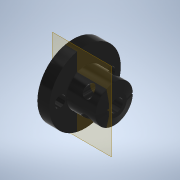
# Autodesk Inventor part: Hub
Saved by Autodesk Inventor 2022 (Build 260153000, 153)
## iProperties
Created: 2022-07-25
Part Number: Hub
Material: Stainless Steel
Document SubType Name: Modeling
Designer: Nathan Cai
Density: 8 g/cm^3
Appearance: Smooth - Black
Author: Nathan Cai
Autodesk Inventor part; units mm, degrees
ref_plane "YZ Plane" through (0, 0, 0) normal (1, 0, 0) x (0, 1, 0)
ref_plane "XZ Plane" through (0, 0, 0) normal (0, 1, 0) x (-1, 0, 0)
sketch "Sketch1" plane through (0, 0, 0) normal (0, 0, 1) x (1, 0, 0)
  line L0 (0, 0) -> (17.145, 0)
  line L1 (0, 0) -> (3.175, 0)
  line L2 (3.175, 0) -> (3.175, 3.175)
  line L3 (3.175, 3.175) -> (0, 3.175)
  line L4 (0, 3.175) -> (0, 0)
  line L5 (3.175, 0) -> (6.985, 0)
  line L6 (6.985, 0) -> (6.985, 11.43)
  line L7 (6.985, 11.43) -> (3.175, 11.43)
  line L8 (3.175, 11.43) -> (3.175, 0)
  line L9 (6.985, 0) -> (17.145, 0)
  line L10 (17.145, 0) -> (17.145, 5.9881)
  line L11 (17.145, 5.9881) -> (6.985, 5.9881)
  line L12 (6.985, 5.9881) -> (6.985, 0)
  line L13 (17.145, 0) -> (10.795, 0)
  line L14 (10.795, 0) -> (10.795, 2)
  line L15 (10.795, 2) -> (17.145, 2)
  line L16 (17.145, 2) -> (17.145, 0)
  line L17 (16.3449, 5.9881) -> (17.145, 3.175)
  point P0 (6.985, 5.9881)
  dimension "d0" = 17.145
  dimension "d1" = 3.175
  dimension "d2" = 3.175
  dimension "d3" = 3.81
  dimension "d4" = 11.43
  dimension "d5" = 10.16
  dimension "d6" = 5.9881
  dimension "d7" = 6.35
  dimension "d8" = 2
  dimension "d10" = 3.175
  dimension "d11" = 9.3599
  constraints: 36 end point, 8 parallel, 5 horizontal, 4 perpendicular, 2 point on line
  measures "d0" distance of L0.start L0.end
  measures "d1" distance of L3.end L2.end
  measures "d2" distance of L2.end L1.end
  measures "d3" distance of L7.end L6.end
  measures "d4" distance of L6.end L5.end
  measures "d5" distance of L11.end L10.end
  measures "d6" distance of L10.end L9.end
  measures "d7" distance of L14.end L15.end
  measures "d8" distance of L13.end L14.end
  measures "d10" distance of L0.end L17.end
  measures "d11" distance from line of L17.start L6
revolve "Revolution1" add sketch "Sketch1" angle 360 about axis through (0, 0, 0) along (1, 0, 0) contours L4 L3 L2 L0 | L2 L8 L7 L6 L0 | L6 L11 L17 L10 L15 L14 L0
fillet "Fillet1" radius 0.1588 5 edges at (6.985, -5.9881, 0) (16.3449, -5.9881, 0) (17.145, -3.175, 0) (3.175, -3.175, 0) (0, -3.175, 0)
sketch "Sketch2" plane through (0, 0, 0) normal (0, 0, 1) x (1, 0, 0)
  line L0 (6.985, -11.43) -> (6.985, 11.43) projected
  line L1 (6.985, 0) -> (12.7, 0) construction
  line L2 (12.7, 0) -> (12.7, 3.81) construction
  circle A0 centre (12.7, 3.81) radius 1.5
  circle A1 centre (12.7, -3.81) radius 1.5
  point P0 (0, 0)
  dimension "d13" = 5.715
  dimension "d14" = 3.81
  dimension "d15" = 3
  constraints: 4 end point, 2 centre point, 1 coincident, 1 horizontal, 1 midpoint, 1 perpendicular, 1 symmetric about line, 1 other
  measures "d13" distance of L1.start L1.end
  measures "d14" distance of L1.end L2.end
  measures "d15" diameter of A0
extrude "Extrusion1" cut sketch "Sketch2" along normal through all both and the other way through all
sketch "Sketch3" plane through (0, 0, 0) normal (0, 1, 0) x (-1, 0, 0)
  line L0 (-7.1437, -5.9881) -> (-7.1437, 5.9881) projected
  line L1 (-7.1437, 5.9881) -> (-19.8438, 5.988)
  line L2 (-19.8438, 5.988) -> (-19.8437, -5.9881)
  line L3 (-19.8437, -5.9881) -> (-7.1437, -5.9881)
  line L4 (-7.1437, -5.9881) -> (-7.1437, 5.9881)
  point P0 (0, 0)
  dimension "d18" = 12.7
  constraints: 8 end point, 2 parallel, 1 horizontal, 1 perpendicular, 1 point on line
  measures "d18" distance between parallel lines of L0 L2
extrude "Extrusion2" cut sketch "Sketch3" along normal mid plane 0.635
ref_plane "Work Plane1" through (0, 0, 2.54) normal (0, 0, 1) x (1, 0, 0)
sketch "Sketch4" plane through (0, 0, 2.54) normal (0, 0, 1) x (1, 0, 0)
  circle A0 centre (12.7, -3.81) radius 2
  line L0 (6.985, -11.43) -> (6.985, 11.43) projected
  line L1 (16.225, -0.3175) -> (7.1437, -0.3175) projected
  point P0 (0, 0)
  point P1 (0, 0)
  dimension "d22" = 4
  dimension "d23" = 5.715
  dimension "d25" = 3.81
  constraints: 1 centre point, 1 coincident
  measures "d22" diameter of A0
  measures "d23" distance from line of L0 A0.centre
  measures "d25" vertical distance of point (0, 0) A0.centre
extrude "Extrusion3" cut sketch "Sketch4" along normal through all
pattern_circular "Circular Pattern1" count 2 over 360 about axis through (13.97, 0, 0) along (1, 0, 0) of "Extrusion3"
sketch "Sketch5" plane through (3.175, 0, 0) normal (-1, 0, 0) x (0, 0, 1)
  circle A0 centre (0, 0) radius 7.9375 construction
  circle A1 centre (7.9375, 0) radius 1.7526
  circle A2 centre (-7.9375, 0) radius 1.7526
  dimension "d31" = 15.875
  dimension "d32" = 3.5052
  dimension "d33" = 3.5052
  constraints: 3 centre point, 2 point on circle, 1 coincident
  measures "d31" diameter of A0
  measures "d32" diameter of A1
  measures "d33" diameter of A2
extrude "Extrusion4" cut sketch "Sketch5" against normal through all
body "Solid1"
